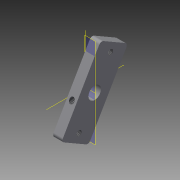
# Autodesk Inventor part: spring_arm
Saved by Autodesk Inventor 2015 (Build 190159000, 159)
## iProperties
Created: 2015-09-03
Part Number: spring_arm
Material: Generic
Description: insert part description/title
Document SubType Name: Modeling
Designer: francis
Density: 1 g/cm^3
Appearance: Default
Author: francis
Part Category: insert part category here and press enter to fill value
Autodesk Inventor part; units mm, degrees
ref_plane "YZ Plane" through (0, 0, 0) normal (1, 0, 0) x (0, 1, 0)
ref_plane "XY Plane" through (0, 0, 0) normal (0, 0, 1) x (1, 0, 0)
sketch "Sketch1" plane through (0, 0, 0) normal (1, 0, 0) x (0, 1, 0)
  line L0 (-2.8397, -24.9186) -> (20.1603, 14.9186)
  line L1 (19.4282, 17.6506) -> (5.5718, 25.6506)
  line L2 (2.8397, 24.9186) -> (-20.1603, -14.9186)
  line L3 (-19.4282, -17.6506) -> (-5.5718, -25.6506)
  line L4 (8.6603, -5) -> (-8.6603, 5) construction
  arc A0 (20.1603, 14.9186) -> (19.4282, 17.6506) centre (18.4282, 15.9186) ccw
  arc A1 (5.5718, 25.6506) -> (2.8397, 24.9186) centre (4.5718, 23.9186) ccw
  arc A2 (-20.1603, -14.9186) -> (-19.4282, -17.6506) centre (-18.4282, -15.9186) ccw
  arc A3 (-5.5718, -25.6506) -> (-2.8397, -24.9186) centre (-4.5718, -23.9186) ccw
  line L5 (-29.1033, 0) -> (29.5375, 0) construction
  line L6 (0, -37.3109) -> (0, 37.3109) construction
  point P0 (0, 0)
  point P1 (-3.8397, -26.6506)
  point P2 (21.1603, 16.6506)
  point P3 (3.8397, 26.6506)
  dimension "d1" = 20
  dimension "d2" = 50
  dimension "d3" = 2
  dimension "d4" = 60
  constraints: 10 end point, 8 point on circle, 8 tangent, 6 point on line, 4 centre point, 3 equal radius, 3 midpoint, 3 perpendicular
  measures "d1" distance of point (21.16, 16.651) point (3.84, 26.651)
  measures "d2" distance of point (-3.84, -26.651) point (21.16, 16.651)
  measures "d3" radius of A0
  measures "d4" angle of L5 L2
extrude "Extrusion1" add sketch "Sketch1" along normal blind 6
sketch "Sketch2" plane through (0, 0, 0) normal (-1, 0, 0) x (0, 0, 1)
  point P0 (0, 0)
hole "Hole1" at (0, 0, 0) direction (1, 0, 0) diameter 8 end through all
sketch "Sketch3" plane through (0, 0, 0) normal (0, 1, 0) x (-1, 0, 0)
  line L0 (-6, -24.9186) -> (-6, 14.9186) construction
  line L1 (0, 14.9186) -> (0, -24.9186) construction
  line L2 (1.2, 0) -> (-7.2, 0) construction
  line L3 (0, 0) -> (-6, 0) construction
  point P0 (-3, 0)
  point P1 (-3, 0)
  constraints: 2 end point, 2 point on line, 1 coincident, 1 midpoint
hole "Hole2" at (3, 0, 0) at (3, 0, 0) direction (0, -1, 0) diameter 3.242 end through all thread size "M4x0.7" class "6H" standard "ISO Metric profile"
sketch "Sketch4" plane through (0, 0, 0) normal (-1, 0, 0) x (0, 0, 1)
  circle A0 centre (0, 0) radius 4 construction
  line L0 (14.9186, 20.1603) -> (-24.9186, -2.8397) construction
  arc A1 (-24.9186, -2.8397) -> (-25.6506, -5.5718) centre (-23.9186, -4.5718) ccw construction
  line L1 (-25.6506, -5.5718) -> (-17.6506, -19.4282) construction
  arc A2 (-17.6506, -19.4282) -> (-14.9186, -20.1603) centre (-15.9186, -18.4282) ccw construction
  line L2 (-14.9186, -20.1603) -> (24.9186, 2.8397) construction
  arc A3 (24.9186, 2.8397) -> (25.6506, 5.5718) centre (23.9186, 4.5718) ccw construction
  line L3 (25.6506, 5.5718) -> (17.6506, 19.4282) construction
  arc A4 (17.6506, 19.4282) -> (14.9186, 20.1603) centre (15.9186, 18.4282) ccw construction
  line L4 (-26.825, -15.4874) -> (32.6029, 18.8233) construction
  line L5 (14.9186, 20.1603) -> (-24.9186, -2.8397) construction
  point P0 (17.3205, 10)
  point P1 (-17.3205, -10)
  dimension "d21" = 20
  dimension "d22" = 20
  constraints: 3 point on line, 2 end point, 1 parallel
  measures "d21" distance of point (0, 0) point (17.321, 10)
  measures "d22" distance of point (0, 0) point (-17.321, -10)
hole "Hole3" at (0, 10, 17.3205) at (0, -10, -17.3205) direction (1, 0, 0) diameter 3.242 end through all thread size "M4x0.7" class "6H" standard "ISO Metric profile"
body "Solid1"
